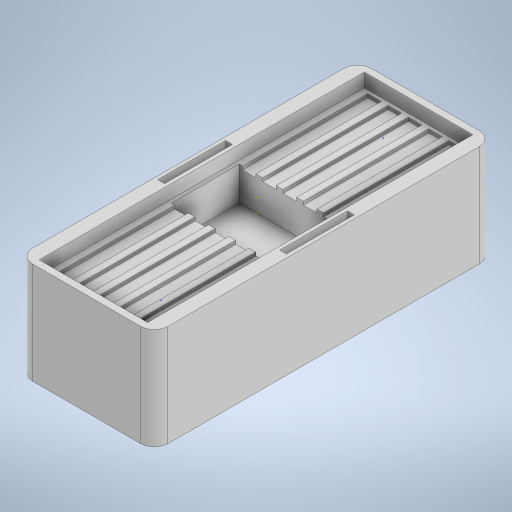
# Autodesk Inventor part: Nadelbox
Saved by Autodesk Inventor 2023.1 (Build 271208000, 208)
## iProperties
Created: 2022-08-08
Part Number: Nadelbox
Material: Generisch
Document SubType Name: Modeling
Designer: schwa
Density: 1 g/cm^3
Appearance: Vorgabe
Author: schwa
Autodesk Inventor part; units mm, degrees
ref_plane "YZ Plane" through (0, 0, 0) normal (1, 0, 0) x (0, 1, 0)
ref_plane "XZ Plane" through (0, 0, 0) normal (0, 1, 0) x (-1, 0, 0)
ref_plane "XY Plane" through (0, 0, 0) normal (0, 0, 1) x (1, 0, 0)
sketch "Skizze1" plane through (0, 0, 0) normal (0, 1, 0) x (-1, 0, 0)
  line L0 (10, 25) -> (-10, 25)
  line L1 (-10, 25) -> (-10, -25)
  line L2 (-10, -25) -> (10, -25)
  line L3 (10, -25) -> (10, 25)
  point P0 (0, 0)
  dimension "d0" = 50
  dimension "d1" = 20
  dimension "d20" = 10
  dimension "d21" = 25
  constraints: 8 end point, 2 parallel, 1 horizontal, 1 perpendicular
  measures "d0" distance of L2.end L0.start
  measures "d1" distance between parallel lines of L1 L3
  measures "d20" distance from line of L3 point (0, 0)
  measures "d21" distance from line of L0 point (0, 0)
extrude "Extrusion1" add sketch "Skizze1" along normal blind 15
sketch "Skizze3" plane through (0, 15, 0) normal (0, 1, 0) x (1, 0, 0)
  line L0 (-8, 24) -> (8, 24)
  line L1 (8, 24) -> (8, -24)
  line L2 (8, -24) -> (-8, -24)
  line L3 (-8, -24) -> (-8, 24)
  line L4 (10, 25) -> (-10, 25) projected
  line L5 (-10, -25) -> (10, -25) projected
  line L6 (10, -25) -> (10, 25) projected
  line L7 (-10, 25) -> (-10, -25) projected
  point P0 (0, 0)
  dimension "d4" = 1
  dimension "d5" = 1
  dimension "d6" = 2
  dimension "d7" = 2
  constraints: 8 end point, 2 parallel, 1 horizontal, 1 perpendicular
  measures "d4" distance between parallel lines of L4 L0
  measures "d5" distance between parallel lines of L2 L5
  measures "d6" distance between parallel lines of L1 L6
  measures "d7" distance between parallel lines of L7 L3
extrude "Extrusion2" cut sketch "Skizze3" against normal blind 2 contours L0 L1 L2 L3
sketch "Skizze4" plane through (0, 13, 0) normal (0, 1, 0) x (1, 0, 0)
  line L0 (-1, 23.5) -> (1, 23.5)
  line L1 (1, 23.5) -> (1, -23.5)
  line L2 (1, -23.5) -> (-1, -23.5)
  line L3 (-1, -23.5) -> (-1, 23.5)
  line L4 (-8, 24) -> (8, 24) projected
  line L5 (8, -24) -> (-8, -24) projected
  line L6 (2, 23.5) -> (4, 23.5)
  line L7 (4, 23.5) -> (4, -23.5)
  line L8 (4, -23.5) -> (2, -23.5)
  line L9 (2, -23.5) -> (2, 23.5)
  line L10 (-7, 23.5) -> (-5, 23.5)
  line L11 (-5, 23.5) -> (-5, -23.5)
  line L12 (-5, -23.5) -> (-7, -23.5)
  line L13 (-7, -23.5) -> (-7, 23.5)
  line L14 (-4, 23.5) -> (-2, 23.5)
  line L15 (-2, 23.5) -> (-2, -23.5)
  line L16 (-2, -23.5) -> (-4, -23.5)
  line L17 (-4, -23.5) -> (-4, 23.5)
  line L18 (5, 23.5) -> (7, 23.5)
  line L19 (7, 23.5) -> (7, -23.5)
  line L20 (7, -23.5) -> (5, -23.5)
  line L21 (5, -23.5) -> (5, 23.5)
  line L22 (-8, -24) -> (-8, 24) projected
  line L23 (8, 24) -> (8, -24) projected
  point P0 (0, 0)
  point P1 (0, -23.5)
  point P2 (0, -24)
  point P3 (6, 23.5)
  dimension "d10" = 2
  dimension "d11" = 0.5
  dimension "d12" = 0.5
  dimension "d33" = 2
  dimension "d34" = 2
  dimension "d35" = 2
  dimension "d36" = 2
  dimension "d37" = 1
  dimension "d38" = 1
  dimension "d39" = 1
  dimension "d40" = 1
  dimension "d41" = 1
  dimension "d42" = 1
  dimension "d50" = 47
  dimension "d51" = 0.5
  dimension "d52" = 0.5
  dimension "d53" = 0.5
  dimension "d54" = 0.5
  dimension "d55" = 47
  constraints: 40 end point, 10 parallel, 5 horizontal, 5 perpendicular, 3 midpoint
  measures "d10" distance of L1.end L2.end
  measures "d11" distance between parallel lines of L4 L0
  measures "d12" distance of point (0, -23.5) point (0, -24)
  measures "d33" distance of L7.end L8.end
  measures "d34" distance of L11.end L13.start
  measures "d35" distance of L15.end L17.start
  measures "d36" distance of L19.end L21.start
  measures "d37" distance between parallel lines of L7 L21
  measures "d38" distance between parallel lines of L1 L9
  measures "d39" distance between parallel lines of L15 L3
  measures "d40" distance between parallel lines of L11 L17
  measures "d41" distance between parallel lines of L22 L13
  measures "d42" distance between parallel lines of L23 L19
  measures "d50" distance between parallel lines of L10 L12
  measures "d51" distance between parallel lines of L5 L12
  measures "d52" distance between parallel lines of L4 L6
  measures "d53" distance between parallel lines of L4 L14
  measures "d54" distance from line of L4 point (6, 23.5)
  measures "d55" distance of L14.start L17.start
sketch "Skizze5" plane through (0, 0, 0) normal (1, 0, 0) x (0, 1, 0)
  point P0 (0, 0)
extrude "Extrusion3" cut sketch "Skizze4" against normal blind 0.5 contours L0 L1 L2 L3 | L6 L7 L8 L9 | L10 L11 L12 L13 | L14 L15 L16 L17 | L18 L19 L20 L21
sketch "Skizze6" plane through (0, 13, 0) normal (0, 1, 0) x (1, 0, 0)
  line L0 (8, 24) -> (8, -24) projected
  point P0 (0, 0)
  point P1 (4.1748, -18.2105)
  point P2 (-0.1937, 19)
  point P3 (8, 0)
  constraints: 1 midpoint
sketch "Skizze8" plane through (0, 15, 0) normal (0, 1, 0) x (1, 0, 0)
  point P0 (0, 0)
sketch "Skizze9" plane through (0, 15, 0) normal (0, 1, 0) x (1, 0, 0)
  line L0 (9.5, 5) -> (8.5, 5)
  line L1 (8.5, 5) -> (8.5, -5)
  line L2 (8.5, -5) -> (9.5, -5)
  line L3 (9.5, -5) -> (9.5, 5)
  line L4 (8, 24) -> (8, -24) construction
  line L5 (-8.5, -5) -> (-9.5, -5)
  line L6 (-9.5, -5) -> (-9.5, 5)
  line L7 (-9.5, 5) -> (-8.5, 5)
  line L8 (-8.5, 5) -> (-8.5, -5)
  line L9 (-10, 25) -> (-10, -25) projected
  point P0 (0, 0)
  point P1 (9, -5)
  point P2 (9.5, 0)
  dimension "d23" = 10
  dimension "d24" = 0.5
  dimension "d25" = 1
  dimension "d26" = 0
  dimension "d29" = 1
  dimension "d30" = 0.5
  constraints: 16 end point, 4 parallel, 2 horizontal, 2 midpoint, 2 perpendicular
  measures "d23" distance from line of point (9, -5) L0
  measures "d24" distance between parallel lines of L4 L1
  measures "d25" distance between parallel lines of L3 L1
  measures "d26" vertical distance of point (0, 0) point (9.5, 0)
  measures "d29" distance of L6.end L7.end
  measures "d30" distance between parallel lines of L9 L6
extrude "Extrusion5" cut sketch "Skizze9" against normal blind 5
sketch "Skizze10" plane through (0, 13, 0) normal (0, 1, 0) x (1, 0, 0)
  line L0 (-7.5, 5) -> (7.5, 5)
  line L1 (7.5, 5) -> (7.5, -5)
  line L2 (7.5, -5) -> (-7.5, -5)
  line L3 (-7.5, -5) -> (-7.5, 5)
  line L4 (-8, -24) -> (-8, 24) projected
  line L5 (8, 24) -> (8, -24) projected
  line L6 (-8, 24) -> (8, 24) projected
  point P0 (0, 0)
  dimension "d43" = 0.5
  dimension "d44" = 0.5
  dimension "d45" = 10
  dimension "d46" = 19
  constraints: 8 end point, 2 parallel, 1 horizontal, 1 perpendicular
  measures "d43" distance between parallel lines of L4 L3
  measures "d44" distance between parallel lines of L1 L5
  measures "d45" distance between parallel lines of L2 L0
  measures "d46" distance between parallel lines of L6 L0
extrude "Extrusion6" cut sketch "Skizze10" against normal blind 5
fillet "Rundung1" radius 2 4 edges at (10, 7.5, 25) (-10, 7.5, 25) (10, 7.5, -25) (-10, 7.5, -25)
sketch "Skizze11" plane through (0, 0, 0) normal (0, -1, 0) x (1, 0, 0)
  line L0 (-4, 17.5) -> (4, 17.5) construction
  line L1 (4, 17.5) -> (4, -17.5) construction
  line L2 (4, -17.5) -> (-4, -17.5) construction
  line L3 (-4, -17.5) -> (-4, 17.5) construction
  line L4 (10, 23) -> (10, -23) projected
  line L5 (-8, 25) -> (8, 25) projected
  line L6 (-4.6135, 2.2719) -> (-5.0964, 2.2719)
  line L7 (-5.0964, 2.2719) -> (-5.8679, 3.6657)
  line L8 (-5.8679, 3.6657) -> (-5.8679, 2.2719)
  line L9 (-5.8679, 2.2719) -> (-6.3266, 2.2719)
  line L10 (-6.3266, 2.2719) -> (-6.3266, 4.2719)
  line L11 (-6.3266, 4.2719) -> (-5.7107, 4.2719)
  line L12 (-5.7107, 4.2719) -> (-5.0721, 3.126)
  line L13 (-5.0721, 3.126) -> (-5.0721, 4.2719)
  line L14 (-5.0721, 4.2719) -> (-4.6135, 4.2719)
  line L15 (-4.6135, 4.2719) -> (-4.6135, 2.2719)
  spline S0 degree 2 poles (-3.4028, 2.4323) (-3.4514, 2.3918) (-3.5276, 2.327) (-3.5924, 2.2946) knots 0 0 0 1 2 2 2
  spline S1 degree 2 poles (-3.5924, 2.2946) (-3.6556, 2.2638) (-3.7755, 2.2314) (-3.8825, 2.2314) knots 0 0 0 1 2 2 2
  spline S2 degree 2 poles (-3.8825, 2.2314) (-4.0835, 2.2314) (-4.3477, 2.5004) (-4.3477, 2.7046) knots 0 0 0 1 2 2 2
  spline S3 degree 2 poles (-4.3477, 2.7046) (-4.3477, 2.8716) (-4.2131, 3.079) (-4.0867, 3.139) knots 0 0 0 1 2 2 2
  spline S4 degree 2 poles (-4.0867, 3.139) (-3.9587, 3.2006) (-3.6037, 3.2492) (-3.3995, 3.2622) knots 0 0 0 1 2 2 2
  line L16 (-3.3995, 3.2622) -> (-3.3995, 3.2703)
  spline S5 degree 2 poles (-3.3995, 3.2703) (-3.3995, 3.3951) (-3.5843, 3.4907) (-3.769, 3.4907) knots 0 0 0 1 2 2 2
  spline S6 degree 2 poles (-3.769, 3.4907) (-3.8517, 3.4907) (-4.0754, 3.4307) (-4.1807, 3.3837) knots 0 0 0 1 2 2 2
  line L17 (-4.1807, 3.3837) -> (-4.2212, 3.3837)
  line L18 (-4.2212, 3.3837) -> (-4.2212, 3.7484)
  spline S7 degree 2 poles (-4.2212, 3.7484) (-4.1515, 3.7678) (-3.8404, 3.8229) (-3.6815, 3.8229) knots 0 0 0 1 2 2 2
  spline S8 degree 2 poles (-3.6815, 3.8229) (-3.2925, 3.8229) (-2.936, 3.5636) (-2.936, 3.2978) knots 0 0 0 1 2 2 2
  line L19 (-2.936, 3.2978) -> (-2.936, 2.2719)
  line L20 (-2.936, 2.2719) -> (-3.4028, 2.2719)
  line L21 (-3.4028, 2.2719) -> (-3.4028, 2.4323)
  line L22 (-3.4028, 2.6657) -> (-3.4028, 2.9785)
  spline S9 degree 2 poles (-3.4028, 2.9785) (-3.5227, 2.9672) (-3.6702, 2.9493) (-3.7415, 2.9234) knots 0 0 0 1 2 2 2
  spline S10 degree 2 poles (-3.7415, 2.9234) (-3.8047, 2.9023) (-3.8728, 2.8148) (-3.8728, 2.7435) knots 0 0 0 1 2 2 2
  spline S11 degree 2 poles (-3.8728, 2.7435) (-3.8728, 2.6382) (-3.7577, 2.5587) (-3.6459, 2.5587) knots 0 0 0 1 2 2 2
  spline S12 degree 2 poles (-3.6459, 2.5587) (-3.5843, 2.5587) (-3.4546, 2.6155) (-3.4028, 2.6657) knots 0 0 0 1 2 2 2
  line L23 (-1.2164, 2.2719) -> (-1.6864, 2.2719)
  line L24 (-1.6864, 2.2719) -> (-1.6864, 2.4291)
  spline S13 degree 2 poles (-1.6864, 2.4291) (-1.7318, 2.3918) (-1.8485, 2.3059) (-1.8938, 2.2832) knots 0 0 0 1 2 2 2
  spline S14 degree 2 poles (-1.8938, 2.2832) (-1.9489, 2.2573) (-2.0592, 2.2297) (-2.1353, 2.2297) knots 0 0 0 1 2 2 2
  spline S15 degree 2 poles (-2.1353, 2.2297) (-2.393, 2.2297) (-2.6945, 2.6576) (-2.6945, 3.0142) knots 0 0 0 1 2 2 2
  spline S16 degree 2 poles (-2.6945, 3.0142) (-2.6945, 3.2119) (-2.5924, 3.502) (-2.5032, 3.609) knots 0 0 0 1 2 2 2
  spline S17 degree 2 poles (-2.5032, 3.609) (-2.4206, 3.7079) (-2.1872, 3.8213) (-2.0575, 3.8213) knots 0 0 0 1 2 2 2
  spline S18 degree 2 poles (-2.0575, 3.8213) (-1.9392, 3.8213) (-1.7869, 3.7711) (-1.6864, 3.7192) knots 0 0 0 1 2 2 2
  line L25 (-1.6864, 3.7192) -> (-1.6864, 4.361)
  line L26 (-1.6864, 4.361) -> (-1.2164, 4.361)
  line L27 (-1.2164, 4.361) -> (-1.2164, 2.2719)
  line L28 (-1.6864, 2.6868) -> (-1.6864, 3.4275)
  spline S19 degree 2 poles (-1.6864, 3.4275) (-1.7204, 3.4453) (-1.8339, 3.468) (-1.8744, 3.468) knots 0 0 0 1 2 2 2
  spline S20 degree 2 poles (-1.8744, 3.468) (-2.0429, 3.468) (-2.2131, 3.2314) (-2.2131, 3.019) knots 0 0 0 1 2 2 2
  spline S21 degree 2 poles (-2.2131, 3.019) (-2.2131, 2.7954) (-2.077, 2.596) (-1.9263, 2.596) knots 0 0 0 1 2 2 2
  spline S22 degree 2 poles (-1.9263, 2.596) (-1.8647, 2.596) (-1.7382, 2.6446) (-1.6864, 2.6868) knots 0 0 0 1 2 2 2
  spline S23 degree 2 poles (-0.0835, 2.2314) (-0.5113, 2.2314) (-0.9668, 2.6398) (-0.9668, 3.0174) knots 0 0 0 1 2 2 2
  spline S24 degree 2 poles (-0.9668, 3.0174) (-0.9668, 3.387) (-0.5421, 3.8278) (-0.1596, 3.8278) knots 0 0 0 1 2 2 2
  spline S25 degree 2 poles (-0.1596, 3.8278) (0.1856, 3.8278) (0.5357, 3.4534) (0.5357, 3.1066) knots 0 0 0 1 2 2 2
  line L29 (0.5357, 3.1066) -> (0.5357, 2.9364)
  line L30 (0.5357, 2.9364) -> (-0.4968, 2.9364)
  spline S26 degree 2 poles (-0.4968, 2.9364) (-0.4903, 2.831) (-0.4141, 2.6917) (-0.3525, 2.6495) knots 0 0 0 1 2 2 2
  spline S27 degree 2 poles (-0.3525, 2.6495) (-0.2925, 2.6074) (-0.1305, 2.5717) (-0.0348, 2.5717) knots 0 0 0 1 2 2 2
  spline S28 degree 2 poles (-0.0348, 2.5717) (0.0462, 2.5717) (0.205, 2.6074) (0.2715, 2.6382) knots 0 0 0 1 2 2 2
  spline S29 degree 2 poles (0.2715, 2.6382) (0.3298, 2.6625) (0.4271, 2.7224) (0.4579, 2.7451) knots 0 0 0 1 2 2 2
  line L31 (0.4579, 2.7451) -> (0.5081, 2.7451)
  line L32 (0.5081, 2.7451) -> (0.5081, 2.3562)
  spline S30 degree 2 poles (0.5081, 2.3562) (0.4498, 2.3335) (0.3558, 2.2946) (0.2715, 2.2751) knots 0 0 0 1 2 2 2
  spline S31 degree 2 poles (0.2715, 2.2751) (0.1953, 2.254) (0.0332, 2.2314) (-0.0835, 2.2314) knots 0 0 0 1 2 2 2
  spline S32 degree 2 poles (0.0721, 3.22) (0.0689, 3.3691) (-0.0624, 3.5263) (-0.1969, 3.5263) knots 0 0 0 1 2 2 2
  spline S33 degree 2 poles (-0.1969, 3.5263) (-0.3347, 3.5263) (-0.4903, 3.361) (-0.4984, 3.22) knots 0 0 0 1 2 2 2
  line L33 (-0.4984, 3.22) -> (0.0721, 3.22)
  line L34 (1.2472, 2.2719) -> (0.7771, 2.2719)
  line L35 (0.7771, 2.2719) -> (0.7771, 4.361)
  line L36 (0.7771, 4.361) -> (1.2472, 4.361)
  line L37 (1.2472, 4.361) -> (1.2472, 2.2719)
  spline S34 degree 2 poles (3.0851, 3.0466) (3.0851, 2.6868) (2.7204, 2.2427) (2.4498, 2.2427) knots 0 0 0 1 2 2 2
  spline S35 degree 2 poles (2.4498, 2.2427) (2.3379, 2.2427) (2.171, 2.2929) (2.077, 2.3464) knots 0 0 0 1 2 2 2
  line L38 (2.077, 2.3464) -> (2.0575, 2.2719)
  line L39 (2.0575, 2.2719) -> (1.607, 2.2719)
  line L40 (1.607, 2.2719) -> (1.607, 4.361)
  line L41 (1.607, 4.361) -> (2.077, 4.361)
  line L42 (2.077, 4.361) -> (2.077, 3.622)
  spline S36 degree 2 poles (2.077, 3.622) (2.1807, 3.7111) (2.3947, 3.8213) (2.5357, 3.8213) knots 0 0 0 1 2 2 2
  spline S37 degree 2 poles (2.5357, 3.8213) (2.7998, 3.8213) (3.0851, 3.4113) (3.0851, 3.0466) knots 0 0 0 1 2 2 2
  spline S38 degree 2 poles (2.6037, 3.0369) (2.6037, 3.2622) (2.4676, 3.455) (2.325, 3.455) knots 0 0 0 1 2 2 2
  spline S39 degree 2 poles (2.325, 3.455) (2.2618, 3.455) (2.137, 3.4145) (2.077, 3.374) knots 0 0 0 1 2 2 2
  line L43 (2.077, 3.374) -> (2.077, 2.6187)
  spline S40 degree 2 poles (2.077, 2.6187) (2.124, 2.5993) (2.2196, 2.5863) (2.2666, 2.5863) knots 0 0 0 1 2 2 2
  spline S41 degree 2 poles (2.2666, 2.5863) (2.4368, 2.5863) (2.6037, 2.8116) (2.6037, 3.0369) knots 0 0 0 1 2 2 2
  spline S42 degree 2 poles (4.7917, 3.0255) (4.7917, 2.6528) (4.3849, 2.2249) (4.0138, 2.2249) knots 0 0 0 1 2 2 2
  spline S43 degree 2 poles (4.0138, 2.2249) (3.6442, 2.2249) (3.2342, 2.6528) (3.2342, 3.0255) knots 0 0 0 1 2 2 2
  spline S44 degree 2 poles (3.2342, 3.0255) (3.2342, 3.4015) (3.6442, 3.8278) (4.0138, 3.8278) knots 0 0 0 1 2 2 2
  spline S45 degree 2 poles (4.0138, 3.8278) (4.3833, 3.8278) (4.7917, 3.3999) (4.7917, 3.0255) knots 0 0 0 1 2 2 2
  spline S46 degree 2 poles (4.3104, 3.0223) (4.3104, 3.1568) (4.2666, 3.3367) (4.2277, 3.3902) knots 0 0 0 1 2 2 2
  spline S47 degree 2 poles (4.2277, 3.3902) (4.1856, 3.4469) (4.0802, 3.4907) (4.0138, 3.4907) knots 0 0 0 1 2 2 2
  spline S48 degree 2 poles (4.0138, 3.4907) (3.9489, 3.4907) (3.8468, 3.4518) (3.8047, 3.3967) knots 0 0 0 1 2 2 2
  spline S49 degree 2 poles (3.8047, 3.3967) (3.7642, 3.3448) (3.7156, 3.1617) (3.7156, 3.0223) knots 0 0 0 1 2 2 2
  spline S50 degree 2 poles (3.7156, 3.0223) (3.7156, 2.8845) (3.7609, 2.7143) (3.7982, 2.6625) knots 0 0 0 1 2 2 2
  spline S51 degree 2 poles (3.7982, 2.6625) (3.8355, 2.6106) (3.9489, 2.562) (4.017, 2.562) knots 0 0 0 1 2 2 2
  spline S52 degree 2 poles (4.017, 2.562) (4.0737, 2.562) (4.1904, 2.6106) (4.2261, 2.6592) knots 0 0 0 1 2 2 2
  spline S53 degree 2 poles (4.2261, 2.6592) (4.2666, 2.716) (4.3104, 2.8797) (4.3104, 3.0223) knots 0 0 0 1 2 2 2
  line L44 (6.5292, 2.2719) -> (5.9781, 2.2719)
  line L45 (5.9781, 2.2719) -> (5.6912, 2.7046)
  line L46 (5.6912, 2.7046) -> (5.3963, 2.2719)
  line L47 (5.3963, 2.2719) -> (4.8566, 2.2719)
  line L48 (4.8566, 2.2719) -> (5.4125, 3.0271)
  line L49 (5.4125, 3.0271) -> (4.8663, 3.7808)
  line L50 (4.8663, 3.7808) -> (5.4173, 3.7808)
  line L51 (5.4173, 3.7808) -> (5.6994, 3.3562)
  line L52 (5.6994, 3.3562) -> (5.983, 3.7808)
  line L53 (5.983, 3.7808) -> (6.5227, 3.7808)
  line L54 (6.5227, 3.7808) -> (5.9765, 3.0385)
  line L55 (5.9765, 3.0385) -> (6.5292, 2.2719)
  line L56 (-5.0421, 0.4878) -> (-5.5835, -1.0211)
  line L57 (-5.5835, -1.0211) -> (-6.0972, -1.0211)
  line L58 (-6.0972, -1.0211) -> (-6.6337, 0.4878)
  line L59 (-6.6337, 0.4878) -> (-6.1394, 0.4878)
  line L60 (-6.1394, 0.4878) -> (-5.8314, -0.5089)
  line L61 (-5.8314, -0.5089) -> (-5.5267, 0.4878)
  line L62 (-5.5267, 0.4878) -> (-5.0421, 0.4878)
  spline S54 degree 2 poles (-3.4149, -0.2674) (-3.4149, -0.6402) (-3.8217, -1.0681) (-4.1929, -1.0681) knots 0 0 0 1 2 2 2
  spline S55 degree 2 poles (-4.1929, -1.0681) (-4.5624, -1.0681) (-4.9724, -0.6402) (-4.9724, -0.2674) knots 0 0 0 1 2 2 2
  spline S56 degree 2 poles (-4.9724, -0.2674) (-4.9724, 0.1086) (-4.5624, 0.5348) (-4.1929, 0.5348) knots 0 0 0 1 2 2 2
  spline S57 degree 2 poles (-4.1929, 0.5348) (-3.8233, 0.5348) (-3.4149, 0.107) (-3.4149, -0.2674) knots 0 0 0 1 2 2 2
  spline S58 degree 2 poles (-3.8963, -0.2707) (-3.8963, -0.1361) (-3.94, 0.0438) (-3.9789, 0.0972) knots 0 0 0 1 2 2 2
  spline S59 degree 2 poles (-3.9789, 0.0972) (-4.0211, 0.154) (-4.1264, 0.1977) (-4.1929, 0.1977) knots 0 0 0 1 2 2 2
  spline S60 degree 2 poles (-4.1929, 0.1977) (-4.2577, 0.1977) (-4.3598, 0.1588) (-4.4019, 0.1037) knots 0 0 0 1 2 2 2
  spline S61 degree 2 poles (-4.4019, 0.1037) (-4.4425, 0.0519) (-4.4911, -0.1313) (-4.4911, -0.2707) knots 0 0 0 1 2 2 2
  spline S62 degree 2 poles (-4.4911, -0.2707) (-4.4911, -0.4084) (-4.4457, -0.5786) (-4.4084, -0.6305) knots 0 0 0 1 2 2 2
  spline S63 degree 2 poles (-4.4084, -0.6305) (-4.3712, -0.6823) (-4.2577, -0.731) (-4.1896, -0.731) knots 0 0 0 1 2 2 2
  spline S64 degree 2 poles (-4.1896, -0.731) (-4.1329, -0.731) (-4.0162, -0.6823) (-3.9806, -0.6337) knots 0 0 0 1 2 2 2
  spline S65 degree 2 poles (-3.9806, -0.6337) (-3.94, -0.577) (-3.8963, -0.4133) (-3.8963, -0.2707) knots 0 0 0 1 2 2 2
  line L63 (-1.7536, -1.0211) -> (-2.2269, -1.0211)
  line L64 (-2.2269, -1.0211) -> (-2.2269, -0.2739)
  spline S66 degree 2 poles (-2.2269, -0.2739) (-2.2269, -0.1815) (-2.2415, 0) (-2.2609, 0.0421) knots 0 0 0 1 2 2 2
  spline S67 degree 2 poles (-2.2609, 0.0421) (-2.2853, 0.094) (-2.376, 0.1378) (-2.4538, 0.1378) knots 0 0 0 1 2 2 2
  spline S68 degree 2 poles (-2.4538, 0.1378) (-2.5105, 0.1378) (-2.6288, 0.094) (-2.6953, 0.047) knots 0 0 0 1 2 2 2
  line L65 (-2.6953, 0.047) -> (-2.6953, -1.0211)
  line L66 (-2.6953, -1.0211) -> (-3.1653, -1.0211)
  line L67 (-3.1653, -1.0211) -> (-3.1653, 0.4878)
  line L68 (-3.1653, 0.4878) -> (-2.6953, 0.4878)
  line L69 (-2.6953, 0.4878) -> (-2.6953, 0.3209)
  spline S69 degree 2 poles (-2.6953, 0.3209) (-2.5802, 0.4182) (-2.3614, 0.5284) (-2.2285, 0.5284) knots 0 0 0 1 2 2 2
  spline S70 degree 2 poles (-2.2285, 0.5284) (-1.9984, 0.5284) (-1.7536, 0.2366) (-1.7536, -0.0389) knots 0 0 0 1 2 2 2
  line L70 (-1.7536, -0.0389) -> (-1.7536, -1.0211)
  line L71 (0.7666, 0.5981) -> (-0.0729, 0.5981)
  line L72 (-0.0729, 0.5981) -> (-0.0729, 0.2204)
  line L73 (-0.0729, 0.2204) -> (0.7002, 0.2204)
  line L74 (0.7002, 0.2204) -> (0.7002, -0.1605)
  line L75 (0.7002, -0.1605) -> (-0.0729, -0.1605)
  line L76 (-0.0729, -0.1605) -> (-0.0729, -1.0211)
  line L77 (-0.0729, -1.0211) -> (-0.5721, -1.0211)
  line L78 (-0.5721, -1.0211) -> (-0.5721, 0.9789)
  line L79 (-0.5721, 0.9789) -> (0.7666, 0.9789)
  line L80 (0.7666, 0.9789) -> (0.7666, 0.5981)
  spline S71 degree 2 poles (1.7715, -1.0616) (1.3436, -1.0616) (0.8882, -0.6532) (0.8882, -0.2755) knots 0 0 0 1 2 2 2
  spline S72 degree 2 poles (0.8882, -0.2755) (0.8882, 0.094) (1.3128, 0.5348) (1.6953, 0.5348) knots 0 0 0 1 2 2 2
  spline S73 degree 2 poles (1.6953, 0.5348) (2.0405, 0.5348) (2.3906, 0.1605) (2.3906, -0.1864) knots 0 0 0 1 2 2 2
  line L81 (2.3906, -0.1864) -> (2.3906, -0.3566)
  line L82 (2.3906, -0.3566) -> (1.3582, -0.3566)
  spline S74 degree 2 poles (1.3582, -0.3566) (1.3647, -0.4619) (1.4408, -0.6013) (1.5024, -0.6434) knots 0 0 0 1 2 2 2
  spline S75 degree 2 poles (1.5024, -0.6434) (1.5624, -0.6856) (1.7245, -0.7212) (1.8201, -0.7212) knots 0 0 0 1 2 2 2
  spline S76 degree 2 poles (1.8201, -0.7212) (1.9011, -0.7212) (2.06, -0.6856) (2.1264, -0.6548) knots 0 0 0 1 2 2 2
  spline S77 degree 2 poles (2.1264, -0.6548) (2.1848, -0.6305) (2.282, -0.5705) (2.3128, -0.5478) knots 0 0 0 1 2 2 2
  line L83 (2.3128, -0.5478) -> (2.363, -0.5478)
  line L84 (2.363, -0.5478) -> (2.363, -0.9368)
  spline S78 degree 2 poles (2.363, -0.9368) (2.3047, -0.9595) (2.2107, -0.9984) (2.1264, -1.0178) knots 0 0 0 1 2 2 2
  spline S79 degree 2 poles (2.1264, -1.0178) (2.0502, -1.0389) (1.8882, -1.0616) (1.7715, -1.0616) knots 0 0 0 1 2 2 2
  spline S80 degree 2 poles (1.9271, -0.0729) (1.9238, 0.0762) (1.7925, 0.2334) (1.658, 0.2334) knots 0 0 0 1 2 2 2
  spline S81 degree 2 poles (1.658, 0.2334) (1.5203, 0.2334) (1.3647, 0.0681) (1.3566, -0.0729) knots 0 0 0 1 2 2 2
  line L85 (1.3566, -0.0729) -> (1.9271, -0.0729)
  line L86 (3.1021, -1.0211) -> (2.6321, -1.0211)
  line L87 (2.6321, -1.0211) -> (2.6321, 1.0681)
  line L88 (2.6321, 1.0681) -> (3.1021, 1.0681)
  line L89 (3.1021, 1.0681) -> (3.1021, -1.0211)
  line L90 (3.9319, -1.0211) -> (3.4619, -1.0211)
  line L91 (3.4619, -1.0211) -> (3.4619, 0.4878)
  line L92 (3.4619, 0.4878) -> (3.9319, 0.4878)
  line L93 (3.9319, 0.4878) -> (3.9319, -1.0211)
  line L94 (3.9465, 0.7034) -> (3.4489, 0.7034)
  line L95 (3.4489, 0.7034) -> (3.4489, 1.0697)
  line L96 (3.4489, 1.0697) -> (3.9465, 1.0697)
  line L97 (3.9465, 1.0697) -> (3.9465, 0.7034)
  line L98 (5.7796, -1.0211) -> (5.2285, -1.0211)
  line L99 (5.2285, -1.0211) -> (4.9417, -0.5883)
  line L100 (4.9417, -0.5883) -> (4.6467, -1.0211)
  line L101 (4.6467, -1.0211) -> (4.107, -1.0211)
  line L102 (4.107, -1.0211) -> (4.6629, -0.2658)
  line L103 (4.6629, -0.2658) -> (4.1167, 0.4878)
  line L104 (4.1167, 0.4878) -> (4.6677, 0.4878)
  line L105 (4.6677, 0.4878) -> (4.9498, 0.0632)
  line L106 (4.9498, 0.0632) -> (5.2334, 0.4878)
  line L107 (5.2334, 0.4878) -> (5.7731, 0.4878)
  line L108 (5.7731, 0.4878) -> (5.2269, -0.2545)
  line L109 (5.2269, -0.2545) -> (5.7796, -1.0211)
  line L110 (6.5251, -0.4927) -> (6.0551, -1.517)
  line L111 (6.0551, -1.517) -> (5.7682, -1.517)
  line L112 (5.7682, -1.517) -> (6.0324, -0.4927)
  line L113 (6.0324, -0.4927) -> (6.5251, -0.4927)
  spline S82 degree 2 poles (-4.4943, -3.2022) (-4.4943, -3.4566) (-4.6126, -3.8813) (-4.7374, -4.0336) knots 0 0 0 1 2 2 2
  spline S83 degree 2 poles (-4.7374, -4.0336) (-4.8671, -4.1876) (-5.2496, -4.3529) (-5.5284, -4.3529) knots 0 0 0 1 2 2 2
  spline S84 degree 2 poles (-5.5284, -4.3529) (-5.6224, -4.3529) (-5.8266, -4.3286) (-5.8606, -4.3189) knots 0 0 0 1 2 2 2
  line L114 (-5.8606, -4.3189) -> (-5.8606, -3.9267)
  line L115 (-5.8606, -3.9267) -> (-5.8217, -3.9267)
  spline S85 degree 2 poles (-5.8217, -3.9267) (-5.7844, -3.9461) (-5.6451, -3.9882) (-5.5235, -3.9882) knots 0 0 0 1 2 2 2
  spline S86 degree 2 poles (-5.5235, -3.9882) (-5.4246, -3.9882) (-5.2415, -3.9364) (-5.1767, -3.8797) knots 0 0 0 1 2 2 2
  spline S87 degree 2 poles (-5.1767, -3.8797) (-5.107, -3.8197) (-5.0162, -3.643) (-5, -3.5101) knots 0 0 0 1 2 2 2
  spline S88 degree 2 poles (-5, -3.5101) (-5.107, -3.5766) (-5.2917, -3.6479) (-5.4295, -3.6479) knots 0 0 0 1 2 2 2
  spline S89 degree 2 poles (-5.4295, -3.6479) (-5.5316, -3.6479) (-5.7212, -3.5928) (-5.799, -3.5344) knots 0 0 0 1 2 2 2
  spline S90 degree 2 poles (-5.799, -3.5344) (-5.9028, -3.455) (-6.0243, -3.2006) (-6.0243, -2.9996) knots 0 0 0 1 2 2 2
  spline S91 degree 2 poles (-6.0243, -2.9996) (-6.0243, -2.8424) (-5.9173, -2.5782) (-5.8201, -2.481) knots 0 0 0 1 2 2 2
  spline S92 degree 2 poles (-5.8201, -2.481) (-5.7229, -2.3837) (-5.4408, -2.2735) (-5.2674, -2.2735) knots 0 0 0 1 2 2 2
  spline S93 degree 2 poles (-5.2674, -2.2735) (-5.0924, -2.2735) (-4.8217, -2.3707) (-4.7245, -2.4728) knots 0 0 0 1 2 2 2
  spline S94 degree 2 poles (-4.7245, -2.4728) (-4.611, -2.5863) (-4.4943, -2.9461) (-4.4943, -3.2022) knots 0 0 0 1 2 2 2
  spline S95 degree 2 poles (-4.9919, -3.1276) (-4.9919, -2.9639) (-5.047, -2.7532) (-5.0972, -2.6949) knots 0 0 0 1 2 2 2
  spline S96 degree 2 poles (-5.0972, -2.6949) (-5.1313, -2.6511) (-5.2188, -2.6139) (-5.269, -2.6139) knots 0 0 0 1 2 2 2
  spline S97 degree 2 poles (-5.269, -2.6139) (-5.3144, -2.6139) (-5.3987, -2.6495) (-5.4376, -2.6949) knots 0 0 0 1 2 2 2
  spline S98 degree 2 poles (-5.4376, -2.6949) (-5.4716, -2.7338) (-5.5203, -2.8845) (-5.5203, -2.9737) knots 0 0 0 1 2 2 2
  spline S99 degree 2 poles (-5.5203, -2.9737) (-5.5203, -3.0709) (-5.47, -3.1957) (-5.4279, -3.233) knots 0 0 0 1 2 2 2
  spline S100 degree 2 poles (-5.4279, -3.233) (-5.3841, -3.2703) (-5.2755, -3.2994) (-5.2075, -3.2994) knots 0 0 0 1 2 2 2
  spline S101 degree 2 poles (-5.2075, -3.2994) (-5.1507, -3.2994) (-5.0324, -3.2686) (-4.9951, -3.2524) knots 0 0 0 1 2 2 2
  spline S102 degree 2 poles (-4.9951, -3.2524) (-4.9951, -3.2378) (-4.9919, -3.1827) (-4.9919, -3.1276) knots 0 0 0 1 2 2 2
  line L116 (-3.6969, -4.314) -> (-4.1718, -4.314)
  line L117 (-4.1718, -4.314) -> (-4.1718, -3.7857)
  line L118 (-4.1718, -3.7857) -> (-3.6969, -3.7857)
  line L119 (-3.6969, -3.7857) -> (-3.6969, -4.314)
  spline S103 degree 2 poles (-1.8363, -3.7581) (-1.8363, -3.8861) (-1.9433, -4.1082) (-2.0454, -4.1892) knots 0 0 0 1 2 2 2
  spline S104 degree 2 poles (-2.0454, -4.1892) (-2.1475, -4.2703) (-2.4408, -4.361) (-2.6305, -4.361) knots 0 0 0 1 2 2 2
  spline S105 degree 2 poles (-2.6305, -4.361) (-2.8331, -4.361) (-3.1361, -4.2686) (-3.2334, -4.1892) knots 0 0 0 1 2 2 2
  spline S106 degree 2 poles (-3.2334, -4.1892) (-3.329, -4.1098) (-3.4198, -3.8942) (-3.4198, -3.7743) knots 0 0 0 1 2 2 2
  spline S107 degree 2 poles (-3.4198, -3.7743) (-3.4198, -3.6025) (-3.2301, -3.374) (-3.0502, -3.2978) knots 0 0 0 1 2 2 2
  line L120 (-3.0502, -3.2978) -> (-3.0502, -3.2897)
  spline S108 degree 2 poles (-3.0502, -3.2897) (-3.2269, -3.2038) (-3.3663, -2.9591) (-3.3663, -2.8083) knots 0 0 0 1 2 2 2
  spline S109 degree 2 poles (-3.3663, -2.8083) (-3.3663, -2.6981) (-3.269, -2.5053) (-3.1734, -2.4291) knots 0 0 0 1 2 2 2
  spline S110 degree 2 poles (-3.1734, -2.4291) (-3.081, -2.3562) (-2.8006, -2.2686) (-2.6256, -2.2686) knots 0 0 0 1 2 2 2
  spline S111 degree 2 poles (-2.6256, -2.2686) (-2.4408, -2.2686) (-2.1653, -2.3481) (-2.0762, -2.4129) knots 0 0 0 1 2 2 2
  spline S112 degree 2 poles (-2.0762, -2.4129) (-1.9854, -2.4777) (-1.8882, -2.6657) (-1.8882, -2.7743) knots 0 0 0 1 2 2 2
  spline S113 degree 2 poles (-1.8882, -2.7743) (-1.8882, -2.9169) (-2.0535, -3.1455) (-2.2237, -3.2249) knots 0 0 0 1 2 2 2
  line L121 (-2.2237, -3.2249) -> (-2.2237, -3.2314)
  spline S114 degree 2 poles (-2.2237, -3.2314) (-2.0243, -3.3124) (-1.8363, -3.575) (-1.8363, -3.7581) knots 0 0 0 1 2 2 2
  spline S115 degree 2 poles (-2.3323, -3.7792) (-2.3323, -3.6803) (-2.4165, -3.5766) (-2.5527, -3.5101) knots 0 0 0 1 2 2 2
  spline S116 degree 2 poles (-2.5527, -3.5101) (-2.5916, -3.4923) (-2.7391, -3.4356) (-2.7958, -3.4113) knots 0 0 0 1 2 2 2
  spline S117 degree 2 poles (-2.7958, -3.4113) (-2.8476, -3.4631) (-2.9303, -3.6187) (-2.9303, -3.7111) knots 0 0 0 1 2 2 2
  spline S118 degree 2 poles (-2.9303, -3.7111) (-2.9303, -3.8505) (-2.752, -4.0174) (-2.6078, -4.0174) knots 0 0 0 1 2 2 2
  spline S119 degree 2 poles (-2.6078, -4.0174) (-2.5673, -4.0174) (-2.4668, -3.9915) (-2.4279, -3.9656) knots 0 0 0 1 2 2 2
  spline S120 degree 2 poles (-2.4279, -3.9656) (-2.3841, -3.9348) (-2.3323, -3.8505) (-2.3323, -3.7792) knots 0 0 0 1 2 2 2
  spline S121 degree 2 poles (-2.376, -2.8327) (-2.376, -2.7305) (-2.5105, -2.609) (-2.6256, -2.609) knots 0 0 0 1 2 2 2
  spline S122 degree 2 poles (-2.6256, -2.609) (-2.7358, -2.609) (-2.8703, -2.7192) (-2.8703, -2.8002) knots 0 0 0 1 2 2 2
  spline S123 degree 2 poles (-2.8703, -2.8002) (-2.8703, -2.8797) (-2.7893, -2.9785) (-2.7034, -3.019) knots 0 0 0 1 2 2 2
  spline S124 degree 2 poles (-2.7034, -3.019) (-2.6661, -3.0385) (-2.5624, -3.079) (-2.4765, -3.1114) knots 0 0 0 1 2 2 2
  spline S125 degree 2 poles (-2.4765, -3.1114) (-2.4246, -3.0434) (-2.376, -2.9153) (-2.376, -2.8327) knots 0 0 0 1 2 2 2
  line L122 (-1.0859, -4.314) -> (-1.5608, -4.314)
  line L123 (-1.5608, -4.314) -> (-1.5608, -3.7857)
  line L124 (-1.5608, -3.7857) -> (-1.0859, -3.7857)
  line L125 (-1.0859, -3.7857) -> (-1.0859, -4.314)
  line L126 (0.7796, -4.314) -> (-0.6904, -4.314)
  line L127 (-0.6904, -4.314) -> (-0.6904, -3.9882)
  spline S126 degree 2 poles (-0.6904, -3.9882) (-0.5041, -3.8391) (-0.2058, -3.5766) (-0.094, -3.4583) knots 0 0 0 1 2 2 2
  spline S127 degree 2 poles (-0.094, -3.4583) (0.0535, -3.3043) (0.1848, -3.0693) (0.1848, -2.9461) knots 0 0 0 1 2 2 2
  spline S128 degree 2 poles (0.1848, -2.9461) (0.1848, -2.8067) (0.0178, -2.6576) (-0.1313, -2.6576) knots 0 0 0 1 2 2 2
  spline S129 degree 2 poles (-0.1313, -2.6576) (-0.2075, -2.6576) (-0.3436, -2.6949) (-0.4133, -2.7241) knots 0 0 0 1 2 2 2
  spline S130 degree 2 poles (-0.4133, -2.7241) (-0.4814, -2.7549) (-0.5786, -2.8197) (-0.6029, -2.8359) knots 0 0 0 1 2 2 2
  line L128 (-0.6029, -2.8359) -> (-0.6418, -2.8359)
  line L129 (-0.6418, -2.8359) -> (-0.6418, -2.3999)
  spline S131 degree 2 poles (-0.6418, -2.3999) (-0.5575, -2.3594) (-0.1977, -2.2751) (-0.0308, -2.2751) knots 0 0 0 1 2 2 2
  spline S132 degree 2 poles (-0.0308, -2.2751) (0.3258, -2.2751) (0.6921, -2.5928) (0.6921, -2.8797) knots 0 0 0 1 2 2 2
  spline S133 degree 2 poles (0.6921, -2.8797) (0.6921, -3.0563) (0.5251, -3.3967) (0.3323, -3.5912) knots 0 0 0 1 2 2 2
  spline S134 degree 2 poles (0.3323, -3.5912) (0.2107, -3.7111) (-0.0178, -3.8975) (-0.0681, -3.9364) knots 0 0 0 1 2 2 2
  line L130 (-0.0681, -3.9364) -> (0.7796, -3.9364)
  line L131 (0.7796, -3.9364) -> (0.7796, -4.314)
  spline S135 degree 2 poles (2.5057, -3.314) (2.5057, -3.5733) (2.423, -3.9623) (2.3306, -4.0936) knots 0 0 0 1 2 2 2
  spline S136 degree 2 poles (2.3306, -4.0936) (2.2399, -4.2233) (1.9465, -4.3562) (1.7358, -4.3562) knots 0 0 0 1 2 2 2
  spline S137 degree 2 poles (1.7358, -4.3562) (1.5235, -4.3562) (1.2318, -4.2233) (1.1394, -4.0904) knots 0 0 0 1 2 2 2
  spline S138 degree 2 poles (1.1394, -4.0904) (1.047, -3.9591) (0.9643, -3.5733) (0.9643, -3.314) knots 0 0 0 1 2 2 2
  spline S139 degree 2 poles (0.9643, -3.314) (0.9643, -3.0482) (1.047, -2.6722) (1.141, -2.5361) knots 0 0 0 1 2 2 2
  spline S140 degree 2 poles (1.141, -2.5361) (1.235, -2.4032) (1.5316, -2.2735) (1.7358, -2.2735) knots 0 0 0 1 2 2 2
  spline S141 degree 2 poles (1.7358, -2.2735) (1.9514, -2.2735) (2.2399, -2.4096) (2.3323, -2.5442) knots 0 0 0 1 2 2 2
  spline S142 degree 2 poles (2.3323, -2.5442) (2.423, -2.6754) (2.5057, -3.0628) (2.5057, -3.314) knots 0 0 0 1 2 2 2
  spline S143 degree 2 poles (2.0016, -3.314) (2.0016, -2.9429) (1.8801, -2.643) (1.7358, -2.643) knots 0 0 0 1 2 2 2
  spline S144 degree 2 poles (1.7358, -2.643) (1.5916, -2.643) (1.4684, -2.9429) (1.4684, -3.3156) knots 0 0 0 1 2 2 2
  spline S145 degree 2 poles (1.4684, -3.3156) (1.4684, -3.6819) (1.5916, -3.9866) (1.7358, -3.9866) knots 0 0 0 1 2 2 2
  spline S146 degree 2 poles (1.7358, -3.9866) (1.8784, -3.9866) (2.0016, -3.6819) (2.0016, -3.314) knots 0 0 0 1 2 2 2
  line L132 (4.2836, -4.314) -> (2.8136, -4.314)
  line L133 (2.8136, -4.314) -> (2.8136, -3.9882)
  spline S147 degree 2 poles (2.8136, -3.9882) (3, -3.8391) (3.2982, -3.5766) (3.41, -3.4583) knots 0 0 0 1 2 2 2
  spline S148 degree 2 poles (3.41, -3.4583) (3.5575, -3.3043) (3.6888, -3.0693) (3.6888, -2.9461) knots 0 0 0 1 2 2 2
  spline S149 degree 2 poles (3.6888, -2.9461) (3.6888, -2.8067) (3.5219, -2.6576) (3.3728, -2.6576) knots 0 0 0 1 2 2 2
  spline S150 degree 2 poles (3.3728, -2.6576) (3.2966, -2.6576) (3.1605, -2.6949) (3.0908, -2.7241) knots 0 0 0 1 2 2 2
  spline S151 degree 2 poles (3.0908, -2.7241) (3.0227, -2.7549) (2.9254, -2.8197) (2.9011, -2.8359) knots 0 0 0 1 2 2 2
  line L134 (2.9011, -2.8359) -> (2.8622, -2.8359)
  line L135 (2.8622, -2.8359) -> (2.8622, -2.3999)
  spline S152 degree 2 poles (2.8622, -2.3999) (2.9465, -2.3594) (3.3063, -2.2751) (3.4733, -2.2751) knots 0 0 0 1 2 2 2
  spline S153 degree 2 poles (3.4733, -2.2751) (3.8298, -2.2751) (4.1961, -2.5928) (4.1961, -2.8797) knots 0 0 0 1 2 2 2
  spline S154 degree 2 poles (4.1961, -2.8797) (4.1961, -3.0563) (4.0292, -3.3967) (3.8363, -3.5912) knots 0 0 0 1 2 2 2
  spline S155 degree 2 poles (3.8363, -3.5912) (3.7147, -3.7111) (3.4862, -3.8975) (3.436, -3.9364) knots 0 0 0 1 2 2 2
  line L136 (3.436, -3.9364) -> (4.2836, -3.9364)
  line L137 (4.2836, -3.9364) -> (4.2836, -4.314)
  line L138 (6.0357, -4.314) -> (4.5656, -4.314)
  line L139 (4.5656, -4.314) -> (4.5656, -3.9882)
  spline S156 degree 2 poles (4.5656, -3.9882) (4.752, -3.8391) (5.0502, -3.5766) (5.1621, -3.4583) knots 0 0 0 1 2 2 2
  spline S157 degree 2 poles (5.1621, -3.4583) (5.3096, -3.3043) (5.4408, -3.0693) (5.4408, -2.9461) knots 0 0 0 1 2 2 2
  spline S158 degree 2 poles (5.4408, -2.9461) (5.4408, -2.8067) (5.2739, -2.6576) (5.1248, -2.6576) knots 0 0 0 1 2 2 2
  spline S159 degree 2 poles (5.1248, -2.6576) (5.0486, -2.6576) (4.9125, -2.6949) (4.8428, -2.7241) knots 0 0 0 1 2 2 2
  spline S160 degree 2 poles (4.8428, -2.7241) (4.7747, -2.7549) (4.6775, -2.8197) (4.6532, -2.8359) knots 0 0 0 1 2 2 2
  line L140 (4.6532, -2.8359) -> (4.6143, -2.8359)
  line L141 (4.6143, -2.8359) -> (4.6143, -2.3999)
  spline S161 degree 2 poles (4.6143, -2.3999) (4.6985, -2.3594) (5.0583, -2.2751) (5.2253, -2.2751) knots 0 0 0 1 2 2 2
  spline S162 degree 2 poles (5.2253, -2.2751) (5.5818, -2.2751) (5.9481, -2.5928) (5.9481, -2.8797) knots 0 0 0 1 2 2 2
  spline S163 degree 2 poles (5.9481, -2.8797) (5.9481, -3.0563) (5.7812, -3.3967) (5.5883, -3.5912) knots 0 0 0 1 2 2 2
  spline S164 degree 2 poles (5.5883, -3.5912) (5.4668, -3.7111) (5.2382, -3.8975) (5.188, -3.9364) knots 0 0 0 1 2 2 2
  line L142 (5.188, -3.9364) -> (6.0357, -3.9364)
  line L143 (6.0357, -3.9364) -> (6.0357, -4.314)
  point P0 (0, 0)
  dimension "d56" = 6
  dimension "d57" = 7.5
  dimension "d58" = 35
  dimension "d59" = 8
  constraints: 2 other
  measures "d56" distance between parallel lines of L4 L1
  measures "d57" distance between parallel lines of L5 L0
  measures "d58" distance between parallel lines of L2 L0
  measures "d59" distance between parallel lines of L3 L1
emboss "Prägen1" sketch "Skizze11" operation cut depth 1 direction (0, 1, 0)
